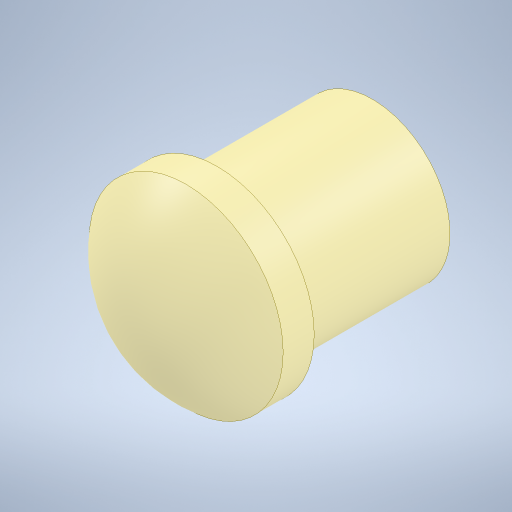
# Autodesk Inventor part: Filler Cap
Saved by Autodesk Inventor 2024 (Build 280153000, 153)
## iProperties
Created: 2021-04-21
Part Number: Filler Cap
Material: Nylon, molybdenum disulphide
Document SubType Name: Modeling
Designer: SauliusD
Density: 1.13 g/cm^3
Appearance: Nylon 6
Author: SauliusD
Autodesk Inventor part; units mm, degrees
ref_plane "YZ Plane" through (0, 0, 0) normal (1, 0, 0) x (0, 1, 0)
ref_plane "XZ Plane" through (0, 0, 0) normal (0, 1, 0) x (-1, 0, 0)
ref_plane "XY Plane" through (0, 0, 0) normal (0, 0, 1) x (1, 0, 0)
sketch "Sketch1" plane through (0, 0, 0) normal (0, 0, 1) x (1, 0, 0)
  line L0 (0, 0) -> (0, 30)
  line L1 (0, 30) -> (-10, 30)
  line L2 (-10, 30) -> (-10, 10)
  line L3 (-10, 10) -> (-12.5, 10)
  line L4 (-12.5, 10) -> (-12.5, 6)
  arc A0 (-12.5, 6) -> (0, 0) centre (0, 16.0208) ccw
  line L5 (0, 30) -> (-7, 30)
  line L6 (-7, 30) -> (-7, 14)
  line L7 (-7, 14) -> (0, 14)
  line L8 (0, 14) -> (0, 30)
  point P0 (0, 14)
  dimension "d0" = 30
  dimension "d1" = 20
  dimension "d2" = 25
  dimension "d3" = 6
  dimension "d4" = 10
  dimension "d5" = 3
  dimension "d6" = 16
  constraints: 18 end point, 5 perpendicular, 2 parallel, 2 point on circle, 1 centre point, 1 horizontal, 1 point on line, 1 vertical
  measures "d0" distance of L0.start L0.end
  measures "d1" diameter of L2 L0
  measures "d2" diameter of L4 L0
  measures "d3" vertical distance of L0.start L4.end
  measures "d4" distance from line of L0.start L3
  measures "d5" distance between parallel lines of L2 L6
  measures "d6" distance of L5.end L6.end
revolve "Revolution1" add sketch "Sketch1" angle 360 about axis through (0, 0, 0) along (0, 1, 0) contours A0 L4 L3 L2 L1 L6 L7 L0
body "Solid1"
